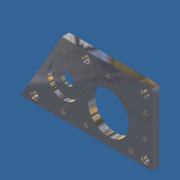
# Autodesk Inventor part: GEARBOX FRONT PLATE
Saved by Autodesk Inventor 2020 (Build 240168000, 168)
## iProperties
Created: 2021-01-14
Part Number: GEARBOX FRONT PLATE
Material: Aluminum 6061
Document SubType Name: Modeling
Designer: lucky
Density: 2.7 g/cm^3
Appearance: Aluminum - Flat
Mass: 38.1624 g
Surface Area: 87.2559 cm^2
Volume: 14.1342 cm^3
Author: lucky
Revision Number: 4
Autodesk Inventor part; units mm, degrees
ref_plane "YZ Plane" through (0, 0, 0) normal (1, 0, 0) x (0, 1, 0)
ref_plane "XZ Plane" through (0, 0, 0) normal (0, 1, 0) x (-1, 0, 0)
ref_plane "XY Plane" through (0, 0, 0) normal (0, 0, 1) x (1, 0, 0)
sketch "MASTER SKETCH" plane through (0, 0, 0) normal (0, 0, 1) x (1, 0, 0)
  circle A0 centre (0, 0) radius 22.86
  circle A1 centre (-31.6504, 3.081) radius 8.89
  circle A2 centre (-31.6504, 3.081) radius 20.32
  circle A3 centre (-60.6627, 6.8802) radius 8.89
  circle A4 centre (-58.2971, 5.0584) radius 6.35
  circle A5 centre (-60.6627, 6.8802) radius 25.4
  circle A6 centre (-58.2971, 5.0584) radius 25.4 construction
  line L0 (-44.0087, 26.0584) -> (-77.3167, -12.298) construction
  line L1 (-68.9445, 30.8921) -> (-52.3809, -17.1317) construction
  line L2 (-85.8186, 10.3933) -> (-36.0162, 0.7394) construction
  circle A7 centre (-44.0087, 26.0584) radius 2
  arc A8 (-68.9445, 30.8921) -> (-69.3394, 27.9326) centre (-44.0087, 26.0584) ccw construction
  arc A9 (-70.9079, 31.2727) -> (-71.334, 28.0802) centre (-44.0087, 26.0584) ccw
  arc A10 (-66.981, 30.5115) -> (-67.3449, 27.785) centre (-44.0087, 26.0584) ccw
  arc A11 (-66.981, 30.5115) -> (-70.9079, 31.2727) centre (-68.9445, 30.8921) ccw
  arc A12 (-71.334, 28.0802) -> (-67.3449, 27.785) centre (-69.3394, 27.9326) ccw
  arc A13 (-85.8186, 10.3933) -> (-83.6914, 5.5953) centre (-44.0087, 26.0584) ccw construction
  arc A14 (-87.6914, 9.6916) -> (-85.469, 4.6787) centre (-44.0087, 26.0584) ccw
  arc A15 (-83.9457, 11.0951) -> (-81.9139, 6.5119) centre (-44.0087, 26.0584) ccw
  arc A16 (-83.9457, 11.0951) -> (-87.6914, 9.6916) centre (-85.8186, 10.3933) ccw
  arc A17 (-85.469, 4.6787) -> (-81.9139, 6.5119) centre (-83.6914, 5.5953) ccw
  arc A18 (-77.3167, -12.298) -> (-72.5856, -15.9416) centre (-44.0087, 26.0584) ccw construction
  arc A19 (-78.6281, -13.8081) -> (-73.7107, -17.5951) centre (-44.0087, 26.0584) ccw
  arc A20 (-76.0054, -10.7879) -> (-71.4605, -14.288) centre (-44.0087, 26.0584) ccw
  arc A21 (-76.0054, -10.7879) -> (-78.6281, -13.8081) centre (-77.3167, -12.298) ccw
  arc A22 (-73.7107, -17.5951) -> (-71.4605, -14.288) centre (-72.5856, -15.9416) ccw
  arc A23 (-52.3809, -17.1317) -> (-47.2548, -17.8157) centre (-44.0087, 26.0584) ccw construction
  arc A24 (-52.7615, -19.0951) -> (-47.4024, -19.8103) centre (-44.0087, 26.0584) ccw
  arc A25 (-52.0003, -15.1682) -> (-47.1072, -15.8212) centre (-44.0087, 26.0584) ccw
  arc A26 (-52.0003, -15.1682) -> (-52.7615, -19.0951) centre (-52.3809, -17.1317) ccw
  arc A27 (-47.4024, -19.8103) -> (-47.1072, -15.8212) centre (-47.2548, -17.8157) ccw
  arc A28 (-36.0162, 0.7394) -> (-33.1003, 1.8522) centre (-44.0087, 26.0584) ccw construction
  arc A29 (-35.4141, -1.1679) -> (-32.2786, 0.0288) centre (-44.0087, 26.0584) ccw
  arc A30 (-36.6183, 2.6466) -> (-33.922, 3.6756) centre (-44.0087, 26.0584) ccw
  arc A31 (-36.6183, 2.6466) -> (-35.4141, -1.1679) centre (-36.0162, 0.7394) ccw
  arc A32 (-32.2786, 0.0288) -> (-33.922, 3.6756) centre (-33.1003, 1.8522) ccw
  line L3 (-91.0627, 30.0584) -> (30.5868, 30.0584)
  line L4 (30.5868, 30.0584) -> (30.5868, -19.9416)
  line L5 (30.5868, -19.9416) -> (-91.0627, -19.9416)
  line L6 (-91.0627, -19.9416) -> (-91.0627, 30.0584)
  circle A33 centre (0, 0) radius 14.2875 construction
  circle A34 centre (25.5868, -14.9416) radius 3
  circle A35 centre (25.5868, 25.0584) radius 3
  circle A36 centre (-51.8755, -14.9416) radius 3
  line L7 (-91.0627, 25.3566) -> (30.5868, 25.3566) construction
  circle A37 centre (-15.8118, 25.0584) radius 3
  line L8 (-58.2971, 5.0584) -> (-60.6627, 6.8802) construction
  line L9 (-52.0979, 13.108) -> (-54.4635, 14.9298)
  line L10 (-66.8619, -1.1693) -> (-64.4963, -2.9911)
  arc A38 (-64.4963, -2.9911) -> (-52.0979, 13.108) centre (-58.2971, 5.0584) ccw
  arc A39 (-54.4635, 14.9298) -> (-66.8619, -1.1693) centre (-60.6627, 6.8802) ccw
  circle A40 centre (0, 0) radius 24.13 construction
  circle A41 centre (-31.6504, 3.081) radius 21.59 construction
  line L11 (-67.7771, -2.3578) -> (-65.4116, -4.1796)
  arc A42 (-65.4116, -4.1796) -> (-51.1827, 14.2964) centre (-58.2971, 5.0584) ccw
  line L12 (-51.1827, 14.2964) -> (-53.5482, 16.1182)
  arc A43 (-53.5482, 16.1182) -> (-67.7771, -2.3578) centre (-60.6627, 6.8802) ccw
  point P0 (-60.0285, -7.7006)
  point P1 (-59.4799, 5.9693)
  dimension "d0" = 45.72
  dimension "d1" = 17.78
  dimension "d2" = 40.64
  dimension "d4" = 17.78
  dimension "d5" = 12.7
  dimension "d6" = 50.8
  dimension "d9" = 50.8
  dimension "d10" = 60
  dimension "d11" = 60
  dimension "d12" = 4
  dimension "d13" = 4
  dimension "d14" = 4
  dimension "d15" = 4
  dimension "d16" = 4
  dimension "d17" = 4
  dimension "d19" = 28.575
  dimension "d28" = 6
  dimension "d29" = 6
  dimension "d30" = 6
  dimension "d39" = 31.8
  dimension "d42" = 29.26
  dimension "d43" = 26.72
  dimension "d70" = 2
  dimension "d73" = 6
  dimension "d84" = 2
  dimension "d85" = 5
  dimension "d89" = 20.32
  dimension "d108" = 1.27
  dimension "d109" = 1.27
  dimension "d110" = 2.5
  dimension "d111" = 2.5
  dimension "d113" = 2.5
  dimension "d114" = 2
  dimension "d129" = 1.5
  dimension "d133" = 2.5
  dimension "d136" = 50
  dimension "d139" = 2
  dimension "d140" = 2.5
  dimension "d141" = 2
  dimension "d142" = 2
  constraints: 70 point on circle, 44 centre point, 28 end point, 24 tangent, 10 coincident, 4 midpoint, 4 parallel, 3 point on line, 2 perpendicular, 1 concentric, 1 horizontal, 1 horizontal alignment, 1 vertical alignment, 3 other
  measures "d0" diameter of A0
  measures "d1" diameter of A1
  measures "d2" diameter of A2
  measures "d4" diameter of A3
  measures "d5" diameter of A4
  measures "d6" diameter of A5
  measures "d9" diameter of A6
  measures "d10" angle of L1 L0
  measures "d11" angle of L2 L1
  measures "d12" diameter of A7
  measures "d13" diameter of A12
  measures "d14" diameter of A17
  measures "d15" diameter of A22
  measures "d16" diameter of A27
  measures "d17" diameter of A32
  measures "d19" diameter of A33
  measures "d28" diameter of A34
  measures "d29" diameter of A35
  measures "d30" diameter of A36
  measures "d39" distance of A0.centre A1.centre
  measures "d42" distance of A1.centre A3.centre
  measures "d43" distance of A1.centre A4.centre
  measures "d70" distance edge to line of A34 L5
  measures "d73" diameter of A37
  measures "d84" distance edge to line of A36 L5
  measures "d85" distance edge to line of A5 L6
  measures "d89" diameter of A39
  measures "d108" radial gap between concentric circles of A0 A40
  measures "d109" radial gap between concentric circles of A2 A41
  measures "d114" distance edge to line of A22 L5
  measures "d129" radial gap between concentric circles of A39 A43
  measures "d136" distance between parallel lines of L5 L3
  measures "d139" distance edge to line of A7 L3
  measures "d141" distance edge to line of A37 L3
  measures "d142" distance edge to line of A34 L4
sketch "Sketch2" plane through (0, 0, 0) normal (0, 0, 1) x (1, 0, 0)
  line L0 (-91.0627, 30.0584) -> (30.5868, 30.0584) projected
  line L1 (-91.0627, -19.9416) -> (-91.0627, 30.0584) projected
  line L2 (30.5868, 30.0584) -> (30.5868, -19.9416) projected
  line L3 (30.5868, -19.9416) -> (-91.0627, -19.9416) projected
  line L4 (-91.0627, 30.0584) -> (30.5868, 30.0584)
  line L5 (30.5868, 30.0584) -> (30.5868, -19.9416)
  line L6 (30.5868, -19.9416) -> (-91.0627, -19.9416)
  line L7 (-91.0627, -19.9416) -> (-91.0627, 30.0584)
  point P0 (0, 0)
  constraints: 8 end point, 2 parallel, 1 horizontal, 1 perpendicular
extrude "Extrusion1" [suppressed]
sketch "Sketch3" plane through (0, 0, 0) normal (0, 0, -1) x (-1, 0, 0)
  arc A0 (47.1072, -15.8212) -> (47.4024, -19.8103) centre (47.2548, -17.8157) ccw projected
  arc A1 (47.1072, -15.8212) -> (52.0003, -15.1682) centre (44.0087, 26.0584) ccw projected
  arc A2 (47.4024, -19.8103) -> (52.7615, -19.0951) centre (44.0087, 26.0584) ccw projected
  arc A3 (52.7615, -19.0951) -> (52.0003, -15.1682) centre (52.3809, -17.1317) ccw projected
  line L0 (91.0627, 30.0584) -> (91.0627, -19.9416) projected
  line L1 (-30.5868, 30.0584) -> (91.0627, 30.0584) projected
  line L2 (-30.5868, -19.9416) -> (-30.5868, 30.0584) projected
  line L3 (91.0627, -19.9416) -> (-30.5868, -19.9416) projected
  arc A4 (71.4605, -14.288) -> (73.7107, -17.5951) centre (72.5856, -15.9416) ccw projected
  arc A5 (73.7107, -17.5951) -> (78.6281, -13.8081) centre (44.0087, 26.0584) ccw projected
  arc A6 (71.4605, -14.288) -> (76.0054, -10.7879) centre (44.0087, 26.0584) ccw projected
  arc A7 (78.6281, -13.8081) -> (76.0054, -10.7879) centre (77.3167, -12.298) ccw projected
  arc A8 (81.9139, 6.5119) -> (83.9457, 11.0951) centre (44.0087, 26.0584) ccw projected
  arc A9 (81.9139, 6.5119) -> (85.469, 4.6787) centre (83.6914, 5.5953) ccw projected
  arc A10 (85.469, 4.6787) -> (87.6914, 9.6916) centre (44.0087, 26.0584) ccw projected
  arc A11 (87.6914, 9.6916) -> (83.9457, 11.0951) centre (85.8186, 10.3933) ccw projected
  arc A12 (71.334, 28.0802) -> (70.9079, 31.2727) centre (44.0087, 26.0584) ccw projected
  arc A13 (67.3449, 27.785) -> (66.981, 30.5115) centre (44.0087, 26.0584) ccw projected
  arc A14 (70.9079, 31.2727) -> (66.981, 30.5115) centre (68.9445, 30.8921) ccw projected
  arc A15 (67.3449, 27.785) -> (71.334, 28.0802) centre (69.3394, 27.9326) ccw projected
  arc A16 (66.8619, -1.1693) -> (54.4635, 14.9298) centre (60.6627, 6.8802) ccw projected
  arc A17 (52.0979, 13.108) -> (64.4963, -2.9911) centre (58.2971, 5.0584) ccw projected
  line L4 (52.0979, 13.108) -> (54.4635, 14.9298) projected
  line L5 (66.8619, -1.1693) -> (64.4963, -2.9911) projected
  point P0 (0, 0)
extrude "Extrusion2" [suppressed]
sketch "Sketch4" plane through (0, 0, 0) normal (0, 0, -1) x (-1, 0, 0)
  circle A0 centre (-25.5868, 25.0584) radius 3 projected
  circle A1 centre (15.8118, 25.0584) radius 3 projected
  circle A2 centre (51.8755, -14.9416) radius 3 projected
  circle A3 centre (-25.5868, -14.9416) radius 3 projected
  point P0 (0, 0)
sketch "Sketch5" plane through (0, 0, 0) normal (0, 0, -1) x (-1, 0, 0)
  circle A0 centre (0, 0) radius 22.86 projected
hole "Hole1" [suppressed]
hole "Hole2" [suppressed]
sketch "Sketch6" plane through (0, 0, 0) normal (0, 0, -1) x (-1, 0, 0)
  line L0 (91.0627, 25.3566) -> (-30.5868, 25.3566) construction
  circle A0 centre (44.0087, 26.0584) radius 2 projected
  point P0 (0, 0)
hole "Hole3" [suppressed]
sketch "Sketch7" plane through (0, 0, 0) normal (0, 0, -1) x (-1, 0, 0)
  circle A0 centre (31.6504, 3.081) radius 20.32 projected
  point P0 (0, 0)
hole "Hole4" [suppressed]
sketch "Sketch8" plane through (0, 0, 0) normal (0, 0, -1) x (-1, 0, 0)
  arc A0 (52.0979, 13.108) -> (64.4963, -2.9911) centre (58.2971, 5.0584) ccw projected
  line L0 (66.8619, -1.1693) -> (64.4963, -2.9911) projected
  arc A1 (66.8619, -1.1693) -> (54.4635, 14.9298) centre (60.6627, 6.8802) ccw projected
  line L1 (52.0979, 13.108) -> (54.4635, 14.9298) projected
  arc A2 (67.7771, -2.3578) -> (53.5482, 16.1182) centre (60.6627, 6.8802) ccw projected
  line L2 (51.1827, 14.2964) -> (53.5482, 16.1182) projected
  line L3 (67.7771, -2.3578) -> (65.4116, -4.1796) projected
  arc A3 (51.1827, 14.2964) -> (65.4116, -4.1796) centre (58.2971, 5.0584) ccw projected
  point P0 (0, 0)
extrude "Extrusion3" [suppressed]
sketch "Sketch11" plane through (0, 0, 0) normal (0, 0, 1) x (1, 0, 0)
  line L0 (30.5868, -19.9416) -> (30.5868, 30.0584) projected
  line L1 (30.5868, 30.0584) -> (30.5868, -19.9416)
  line L2 (30.5868, -19.9416) -> (-61.3292, -19.9416)
  line L3 (-91.0627, -19.9416) -> (30.5868, -19.9416) projected
  line L4 (-61.3292, -19.9416) -> (-32.4617, 30.0584)
  line L5 (30.5868, 30.0584) -> (-91.0627, 30.0584) projected
  line L6 (-32.4617, 30.0584) -> (30.5868, 30.0584)
  circle A0 centre (-44.0087, 26.0584) radius 2 projected
  point P0 (0, 0)
  dimension "d147" = 120
  dimension "d148" = 8
  constraints: 8 end point, 2 point on line, 1 collinear, 1 parallel
  measures "d147" angle of L4 L5
  measures "d148" distance from line of A0.centre L4
extrude "Extrusion5" add sketch "Sketch11" against normal blind 5 contours L2 L4 L5 L0
sketch "Sketch12" plane through (0, 0, 0) normal (0, 0, 1) x (1, 0, 0)
  circle A0 centre (-15.8118, 25.0584) radius 3 projected
  circle A1 centre (25.5868, 25.0584) radius 3 projected
  circle A2 centre (25.5868, -14.9416) radius 3 projected
  circle A3 centre (-51.8755, -14.9416) radius 3 projected
  point P0 (0, 0)
hole "Hole5" at (-15.8118, 25.0584, 0) at (-51.8755, -14.9416, 0) at (25.5868, -14.9416, 0) at (25.5868, 25.0584, 0) direction (0, 0, -1) diameter 4.5 end through all counterbore diameter 6 counterbore depth 1
sketch "Sketch13" plane through (0, 0, 0) normal (0, 0, 1) x (1, 0, 0)
  circle A0 centre (0, 0) radius 14.2875 construction
hole "Hole6" at (0, 0, 0) direction (0, 0, -1) diameter 28.575 end through all
sketch "Sketch14" plane through (0, 0, 0) normal (0, 0, 1) x (1, 0, 0)
  circle A0 centre (-31.6504, 3.081) radius 8.89 projected
  point P0 (0, 0)
hole "Hole7" at (-31.6504, 3.081, 0) direction (0, 0, -1) diameter 8 depth 5 counterbore diameter 22 counterbore depth 3
sketch "Sketch15" plane through (0, 0, -5) normal (0, 0, -1) x (-1, 0, 0)
  circle A0 centre (-25.5868, 25.0584) radius 2.25 projected
  circle A1 centre (-25.5868, -14.9416) radius 2.25 projected
  circle A2 centre (51.8755, -14.9416) radius 2.25 projected
  circle A3 centre (15.8118, 25.0584) radius 2.25 projected
  point P0 (0, 0)
hole "Hole8" at (25.5868, 25.0584, -5) at (-15.8118, 25.0584, -5) at (25.5868, -14.9416, -5) at (-51.8755, -14.9416, -5) direction (0, 0, 1) diameter 4 end through all countersink diameter 8 countersink angle 90
sketch "Sketch16" plane through (0, 0, -5) normal (0, 0, -1) x (-1, 0, 0)
  circle A0 centre (-25.5868, 25.0584) radius 4 construction
  circle A1 centre (-25.5868, -14.9416) radius 4 construction
  circle A2 centre (15.8118, 25.0584) radius 4 construction
  circle A3 centre (51.8755, -14.9416) radius 4 construction
  circle A4 centre (31.6504, 3.081) radius 4 projected
  point P0 (0, 0)
  point P1 (-25.5868, -2.9416)
  point P2 (-25.5868, 13.0584)
  point P3 (15.8118, -14.9416)
  point P4 (0, 22.5584)
  point P5 (-15.5868, -14.9416)
  point P6 (31.6504, -14.9416)
  point P7 (31.6504, 22.5584)
  dimension "d181" = 10
  dimension "d182" = 12
  dimension "d183" = 12
  dimension "d191" = 2.5
  constraints: 7 vertical alignment, 4 horizontal alignment
  measures "d181" distance of point (-15.587, -14.942) A1.centre
  measures "d182" distance of point (-25.587, -2.942) A1.centre
  measures "d183" distance of point (-25.587, 13.058) A0.centre
  measures "d191" vertical distance of point (0, 22.558) A0.centre
hole "Hole9" at (25.5868, -2.9416, -5) at (25.5868, 13.0584, -5) at (-15.8118, -14.9416, -5) at (0, 22.5584, -5) at (15.5868, -14.9416, -5) at (-31.6504, -14.9416, -5) at (-31.6504, 22.5584, -5) direction (0, 0, 1) diameter 3.242 depth 10 thread size "M4x0.7" class "6H" standard "ISO Metric profile"
equation "\"d0\" = SR2PD"
equation "\"d1\" = SR1PD"
equation "\"d2\" = FirstReductionPD"
equation "\"d4\" = Pinion4inPD"
equation "\"d5\" = PinionPD"
equation "\"PinionPD\" = 12.7"
equation "\"FirstReductionPD\" = 40.64"
equation "\"HighGearPD\" = 20.32"
equation "\"LowGearPD\" = 17.78"
equation "\"HighGearDogPD\" = 63.5"
equation "\"LowGearDogPD\" = 76.2"
equation "\"SR1PD\" = 17.78"
equation "\"SR2PD\" = 45.72"
equation "\"Pinion4inPD\" = 17.78"
body "Solid1"
